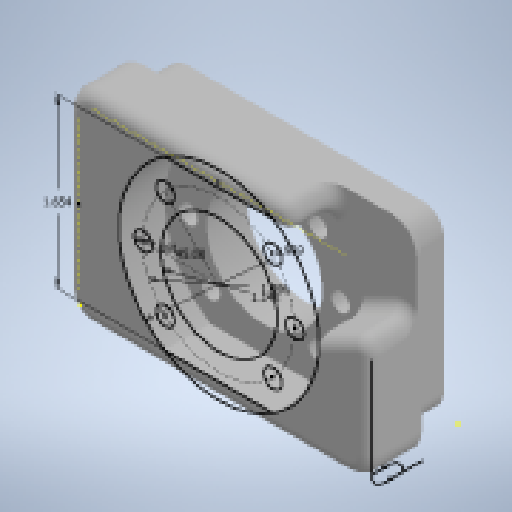
# Autodesk Inventor part: 2x3_Spacer
Saved by Autodesk Inventor 2023 (Build 270158000, 158)
## iProperties
Created: 2022-05-03
Part Number: 2x3_Spacer
Material: Generic
Document SubType Name: Modeling
Designer: plebbb
Density: 1 g/cm^3
Appearance: Default
Mass: 93.191 g
Surface Area: 210.237 cm^2
Volume: 93.191 cm^3
Author: plebbb
Autodesk Inventor part; units mm, degrees
ref_plane "YZ Plane" through (0, 0, 0) normal (1, 0, 0) x (0, 1, 0)
ref_plane "XZ Plane" through (0, 0, 0) normal (0, 1, 0) x (-1, 0, 0)
ref_plane "XY Plane" through (0, 0, 0) normal (0, 0, 1) x (1, 0, 0)
sketch "Sketch1" plane through (0, 0, 0) normal (0, 0, 1) x (1, 0, 0)
  line L0 (5.08, 0) -> (64.135, 0)
  line L1 (69.215, 5.08) -> (69.215, 38.735)
  line L2 (64.135, 43.815) -> (5.08, 43.815)
  line L3 (0, 38.735) -> (0, 5.08)
  arc A0 (5.08, 43.815) -> (0, 38.735) centre (5.08, 38.735) ccw
  arc A1 (0, 5.08) -> (5.08, 0) centre (5.08, 5.08) ccw
  arc A2 (69.215, 38.735) -> (64.135, 43.815) centre (64.135, 38.735) ccw
  arc A3 (64.135, 0) -> (69.215, 5.08) centre (64.135, 5.08) ccw
  point P0 (0, 0)
  point P1 (69.215, 43.815)
  point P2 (69.215, 0)
  point P3 (0, 43.815)
  dimension "d0" = 69.215
  dimension "d1" = 43.815
  dimension "d3" = 5.08
  constraints: 8 end point, 8 point on circle, 8 point on line, 8 tangent, 4 centre point, 3 equal radius, 2 parallel, 1 horizontal, 1 perpendicular
  measures "d0" distance of point (69.215, 43.815) point (0, 43.815)
  measures "d1" distance of point (69.215, 0) point (69.215, 43.815)
  measures "d3" radius of A0
extrude "Extrusion1" add sketch "Sketch1" along normal blind 9
sketch "Sketch2" plane through (0, 0, 9) normal (0, 0, 1) x (1, 0, 0)
  line L0 (2.8575, -3.4925) -> (66.3575, -3.4925)
  line L1 (72.7075, 2.8575) -> (72.7075, 40.9575)
  line L2 (66.3575, 47.3075) -> (2.8575, 47.3075)
  line L3 (-3.4925, 40.9575) -> (-3.4925, 2.8575)
  line L4 (64.135, 43.815) -> (5.08, 43.815) construction
  line L5 (0, 38.735) -> (0, 5.08) construction
  line L6 (5.08, 0) -> (64.135, 0) construction
  line L7 (69.215, 5.08) -> (69.215, 38.735) construction
  arc A0 (2.8575, 47.3075) -> (-3.4925, 40.9575) centre (2.8575, 40.9575) ccw
  arc A1 (-3.4925, 2.8575) -> (2.8575, -3.4925) centre (2.8575, 2.8575) ccw
  arc A2 (66.3575, -3.4925) -> (72.7075, 2.8575) centre (66.3575, 2.8575) ccw
  arc A3 (72.7075, 40.9575) -> (66.3575, 47.3075) centre (66.3575, 40.9575) ccw
  point P0 (0, 0)
  point P1 (72.7075, 47.3075)
  point P2 (72.7075, -3.4925)
  point P3 (-3.4925, 47.3075)
  point P4 (34.6075, 47.3075)
  point P5 (34.6075, 43.815)
  point P6 (69.215, 21.9075)
  point P7 (72.7075, 21.9075)
  dimension "d6" = 76.2
  dimension "d7" = 50.8
  dimension "d8" = 6.35
  constraints: 8 end point, 8 point on circle, 8 tangent, 6 point on line, 4 centre point, 4 midpoint, 3 equal radius, 2 parallel, 1 horizontal, 1 horizontal alignment, 1 perpendicular, 1 vertical alignment
  measures "d6" distance of point (72.707, 47.308) point (-3.493, 47.308)
  measures "d7" distance of point (72.707, -3.493) point (72.707, 47.308)
  measures "d8" radius of A0
extrude "Extrusion2" add sketch "Sketch2" along normal blind 12.7
fillet "Fillet1" radius 3.175 8 edges at (-1.6326, 45.4476, 21.7) (-3.4925, 21.9075, 21.7) (-1.6326, -1.6326, 21.7) (34.6075, -3.4925, 21.7) (70.8476, -1.6326, 21.7) (72.7075, 21.9075, 21.7) (70.8476, 45.4476, 21.7) (34.6075, 47.3075, 21.7)
sketch "Sketch3" plane through (0, 0, 21.7) normal (0, 0, 1) x (1, 0, 0)
  circle A0 centre (34.6075, 21.9075) radius 14.5
  line L0 (-0.3175, 2.8575) -> (-0.3175, 40.9575) construction
  line L1 (2.8575, 44.1325) -> (66.3575, 44.1325) construction
  circle A1 centre (34.6075, 21.9075) radius 19 construction
  circle A2 centre (48.042529, 35.342529) radius 2.3
  circle A3 centre (15.6075, 21.9075) radius 2.3
  circle A4 centre (48.042529, 8.472471) radius 2.3
  circle A5 centre (53.6075, 21.9075) radius 2.3
  circle A6 centre (21.172471, 35.342529) radius 2.3
  circle A7 centre (21.172471, 8.472471) radius 2.3
  line L2 (21.172471, 35.342529) -> (34.6075, 21.9075) construction
  line L3 (34.6075, 21.9075) -> (15.6075, 21.9075) construction
  circle A8 centre (34.6075, 21.9075) radius 25
  line L4 (21.04284, 42.9075) -> (48.17216, 42.9075)
  line L5 (48.17216, 0.9075) -> (21.04284, 0.9075)
  point P0 (0, 0)
  point P1 (34.6075, 44.1325)
  point P2 (-0.3175, 21.9075)
  dimension "d12" = 29
  dimension "d13" = 38
  dimension "d14" = 4.6
  dimension "d15" = 45
  dimension "d28" = 50
  dimension "d29" = 42
  constraints: 10 point on circle, 9 centre point, 8 end point, 5 equal radius, 4 horizontal alignment, 3 vertical alignment, 2 coincident, 2 horizontal, 2 midpoint, 2 parallel
  measures "d12" diameter of A0
  measures "d13" diameter of A1
  measures "d14" diameter of A3
  measures "d15" angle of L3 L2
  measures "d28" diameter of A8
  measures "d29" distance between parallel lines of L5 L4
extrude "Extrusion3" cut sketch "Sketch3" against normal up to surface (21.7 mm away) contours A0 | A2 | A3 | A4 | A5 | A6 | A7
extrude "Extrusion6" cut sketch "Sketch3" against normal blind 11.5 contours A8 L5 L4
sketch "Sketch9" plane through (0, 0, 10.2) normal (0, 0, 1) x (1, 0, 0)
  arc A0 (48.17216, 0.9075) -> (48.17216, 42.9075) centre (34.6075, 21.9075) ccw
  line L0 (34.6075, 21.9075) -> (57.704488, 31.474586)
  line L1 (34.6075, 21.9075) -> (34.6075, 36.491135)
  line L2 (57.704488, 31.474586) -> (68.791043, 36.066787)
  arc A1 (59.606166, 22.165749) -> (50.52263, 41.187247) centre (34.6075, 21.9075) ccw
  line L3 (50.52263, 41.187247) -> (74.194194, 52.980155)
  line L4 (74.194194, 52.980155) -> (83.255211, 34.792237)
  line L5 (83.255211, 34.792237) -> (59.583647, 22.999329)
  arc A2 (48.17216, 0.9075) -> (48.17216, 42.9075) centre (34.6075, 21.9075) ccw
  point P0 (0, 0)
  dimension "d32" = 67.5
  dimension "d33" = 12
  dimension "d35" = 20.32
  constraints: 12 end point, 7 point on circle, 2 perpendicular, 1 centre point, 1 collinear, 1 parallel, 1 vertical
  measures "d32" angle of L0 L1
  measures "d33" distance of L0.end L2.end
  measures "d35" distance of L3.end L4.end
extrude "Extrusion7" cut sketch "Sketch9" along normal blind 25.4
fillet "Fillet2" radius 3.175 8 edges at (56.6651, 44.2474, 10.2) (60.941, 46.3776, 20.7701) (53.4786, 42.6599, 21.7) (62.8076, 47.3075, 14.3625) (64.5581, 25.4775, 21.7) (72.7075, 29.5375, 14.3625) (71.7776, 29.0742, 20.7701) (66.1456, 26.2684, 10.2)
sketch "Sketch10" plane through (72.7075, 2.8575, 9) normal (1, 0, 0) x (0, 0, -1)
  arc A0 (-12.7, -3.175) -> (-9.525, -6.35) centre (-9.525, -3.175) ccw
  line L0 (0, -6.35) -> (-9.525, -6.35)
  line L1 (-12.7, 21.551046) -> (-12.7, 0)
  line L2 (-12.7, -3.175) -> (-12.7, 0)
  arc A1 (-12.7, -3.175) -> (-9.525, -6.35) centre (-9.525, -3.175) ccw
  line L3 (-12.7, -3.175) -> (-12.7, 0)
  line L4 (-12.7, -3.175) -> (-7.9375, -3.175)
  arc A2 (-4.7625, -6.35) -> (-7.9375, -3.175) centre (-7.9375, -6.35) ccw
  point P0 (9, -2.8575)
  constraints: 8 end point, 4 point on circle, 2 centre point, 2 horizontal, 2 vertical, 1 line through centre, 1 midpoint, 1 tangent, 7 other
extrude "Extrusion8" cut sketch "Sketch10" against normal blind 47.625
body "Solid1"
